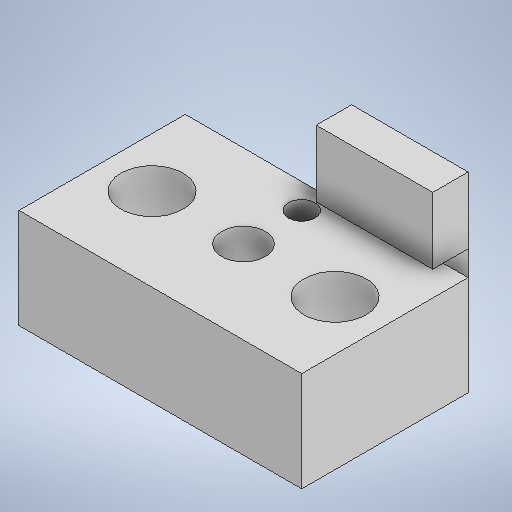
# Autodesk Inventor part: Taster_Schlitten
Saved by Autodesk Inventor 2025 (Build 290162000, 162)
## iProperties
Created: 2026-07-10
Part Number: Taster_Schlitten
Material: Generisch
Document SubType Name: Modeling
Designer: wavid
Mass: 59.1285 g
Surface Area: 172.778 cm^2
Volume: 59.1285 cm^3
Density: 1 g/cm^3
Appearance: Vorgabe
Author: wavid
Autodesk Inventor part; units mm, degrees
ref_plane "YZ Plane" through (0, 0, 0) normal (1, 0, 0) x (0, 1, 0)
sketch "Skizze1" plane through (0, 0, 0) normal (0, 0, 1) x (1, 0, 0)
  line L0 (-34, -20) -> (34, -20)
  line L1 (34, -20) -> (34, 20)
  line L2 (34, 20) -> (-34, 20)
  line L3 (-34, 20) -> (-34, -20)
  constraints: 8 end point, 2 parallel, 1 horizontal, 1 perpendicular
extrude "Extrusion1" add sketch "Skizze1" along normal blind 24
sketch "Skizze2" plane through (0, 0, 0) normal (0, 0, 1) x (1, 0, 0)
  line L0 (0, 20) -> (28, 20)
  line L1 (28, 20) -> (28, 26)
  line L2 (28, 26) -> (0, 26)
  line L3 (0, 26) -> (0, 20)
  constraints: 8 end point, 2 parallel, 1 horizontal, 1 perpendicular
extrude "Extrusion2" add sketch "Skizze2" along normal blind 24 separate body
ref_plane "Arbeitsebene1" through (0, 0, 24) normal (0, 0, 1) x (1, 0, 0)
sketch "Skizze3" plane through (0, 0, 24) normal (0, 0, 1) x (1, 0, 0)
  line L0 (0, 17.5) -> (28, 17.5)
  line L1 (28, 17.5) -> (28, 26)
  line L2 (28, 26) -> (0, 26)
  line L3 (0, 26) -> (0, 17.5)
  constraints: 8 end point, 2 parallel, 1 horizontal, 1 perpendicular
extrude "Extrusion3" add sketch "Skizze3" along normal blind 16 separate body
sketch "Skizze4" plane through (0, 0, 24) normal (0, 0, 1) x (1, 0, 0)
  circle A0 centre (-22, 0) radius 7.5
  constraints: 1 centre point
extrude "Extrusion4" cut sketch "Skizze4" against normal blind 24.2 bodies 1
sketch "Skizze5" plane through (0, 0, 24) normal (0, 0, 1) x (1, 0, 0)
  circle A0 centre (22, 0) radius 7.5
  constraints: 1 centre point
extrude "Extrusion5" cut sketch "Skizze5" against normal blind 24.2 bodies 1
sketch "Skizze6" plane through (0, 0, 24) normal (0, 0, 1) x (1, 0, 0)
  circle A0 centre (0, 0) radius 5.25
  constraints: 1 centre point
extrude "Extrusion6" cut sketch "Skizze6" against normal blind 24.2 bodies 1
sketch "Skizze7" plane through (0, 0, 24) normal (0, 0, 1) x (1, 0, 0)
  circle A0 centre (0, 14) radius 3.2
  constraints: 1 centre point
extrude "Extrusion7" cut sketch "Skizze7" against normal blind 24.2 bodies 1
sketch "Skizze8" plane through (0, 0, 0) normal (0, 0, 1) x (1, 0, 0)
  circle A0 centre (0, 0) radius 11.2
  constraints: 1 centre point
extrude "Extrusion8" cut sketch "Skizze8" along normal blind 4 bodies 1
sketch "Skizze9" plane through (0, 0, 0) normal (0, 0, 1) x (1, 0, 0)
  circle A0 centre (5.6569, 5.6569) radius 1.4
  constraints: 1 centre point
extrude "Extrusion9" cut sketch "Skizze9" along normal blind 8 bodies 1
sketch "Skizze10" plane through (0, 0, 0) normal (0, 0, 1) x (1, 0, 0)
  circle A0 centre (-5.6569, 5.6569) radius 1.4
  constraints: 1 centre point
extrude "Extrusion10" cut sketch "Skizze10" along normal blind 8 bodies 1
sketch "Skizze11" plane through (0, 0, 0) normal (0, 0, 1) x (1, 0, 0)
  circle A0 centre (-5.6569, -5.6569) radius 1.4
  constraints: 1 centre point
extrude "Extrusion11" cut sketch "Skizze11" along normal blind 8 bodies 1
sketch "Skizze12" plane through (0, 0, 0) normal (0, 0, 1) x (1, 0, 0)
  circle A0 centre (5.6569, -5.6569) radius 1.4
  constraints: 1 centre point
extrude "Extrusion12" cut sketch "Skizze12" along normal blind 8 bodies 1
sketch "Skizze13" plane through (0, 0, 0) normal (0, 0, 1) x (1, 0, 0)
  circle A0 centre (0, 14) radius 6.5
  constraints: 1 centre point
extrude "Extrusion13" cut sketch "Skizze13" along normal blind 14 bodies 1
sketch "Skizze14" plane through (0, 0, 0) normal (0, 0, 1) x (1, 0, 0)
  circle A0 centre (-9, 14) radius 1
  constraints: 1 centre point
extrude "Extrusion14" cut sketch "Skizze14" along normal blind 8 bodies 1
sketch "Skizze15" plane through (0, 0, 0) normal (0, 0, 1) x (1, 0, 0)
  circle A0 centre (9, 14) radius 1
  constraints: 1 centre point
extrude "Extrusion15" cut sketch "Skizze15" along normal blind 8 bodies 1
ref_plane "Arbeitsebene2" through (0, 17.5, 0) normal (0, 1, 0) x (-1, 0, 0)
sketch "Skizze16" plane through (0, 17.5, 0) normal (0, 1, 0) x (-1, 0, 0)
  line L0 (1.3, 30) -> (4.5, 30)
  line L1 (4.5, 30) -> (4.5, 38)
  line L2 (4.5, 38) -> (1.3, 38)
  line L3 (1.3, 38) -> (1.3, 30)
  constraints: 8 end point, 2 parallel, 1 horizontal, 1 perpendicular
extrude "Extrusion16" cut sketch "Skizze16" along normal blind 8.7 bodies 1
sketch "Skizze17" plane through (0, 17.5, 0) normal (0, 1, 0) x (-1, 0, 0)
  line L0 (23.5, 30) -> (26.7, 30)
  line L1 (26.7, 30) -> (26.7, 38)
  line L2 (26.7, 38) -> (23.5, 38)
  line L3 (23.5, 38) -> (23.5, 30)
  constraints: 8 end point, 2 parallel, 1 horizontal, 1 perpendicular
extrude "Extrusion17" cut sketch "Skizze17" along normal blind 8.7 bodies 1
